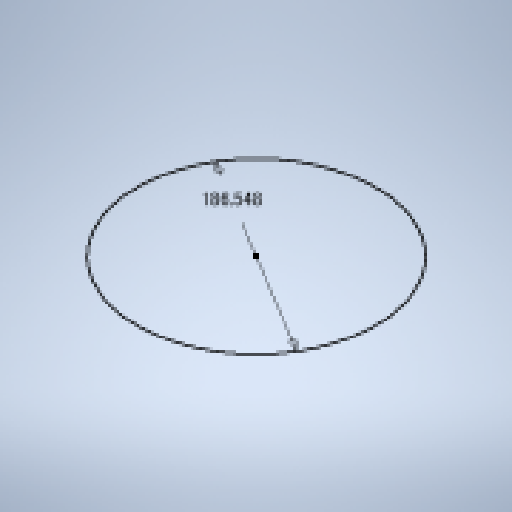
# Autodesk Inventor part: baseplate_R2toR3
Saved by Autodesk Inventor 2024.3 (Build 283343010, 343A)
## iProperties
Created: 2025-05-25
Part Number: baseplate_R2toR3
Material: アルミニウム 6061
Document SubType Name: Modeling
Designer: kshau
Density: 2.7 g/cm^3
Appearance: アルミニウム - フラット
Mass: 150.999 g
Surface Area: 394.685 cm^2
Volume: 55.9256 cm^3
Author: kshau
Autodesk Inventor part; units mm, degrees
ref_plane "YZ Plane" through (0, 0, 0) normal (1, 0, 0) x (0, 1, 0)
ref_plane "XZ Plane" through (0, 0, 0) normal (0, 1, 0) x (-1, 0, 0)
ref_plane "XY Plane" through (0, 0, 0) normal (0, 0, 1) x (1, 0, 0)
sketch "スケッチ1" plane through (0, 0, 0) normal (0, 1, 0) x (-1, 0, 0)
  circle A0 centre (0, 0) radius 86.2565
  circle A1 centre (0, 0) radius 6.25
  dimension "d0" = 172.513
  dimension "d1" = 12.5
  constraints: 2 centre point, 2 coincident
  measures "d0" diameter of A0
  measures "d1" diameter of A1
extrude "押し出し1" add sketch "スケッチ1" along normal blind 3
sketch "スケッチ2" plane through (0, 3, 0) normal (0, 1, 0) x (1, 0, 0)
  circle A0 centre (0, 0) radius 50.75
  point P0 (0, 50.75)
  point P1 (-50.75, 0)
  point P2 (0, -50.75)
  point P3 (50.75, 0)
  dimension "d4" = 101.5
  dimension "d7" = 360
  constraints: 1 coincident, 1 vertical alignment, 7 other
hole "穴1" at (0, 3, -50.75) at (-50.75, 3, 0) at (0, 3, 50.75) at (50.75, 3, 0) direction (0, -1, 0) diameter 4.3 end through all
sketch "スケッチ3" plane through (0, 3, 0) normal (0, 1, 0) x (1, 0, 0)
  line L0 (0, 0) -> (86.2565, 0)
  circle A0 centre (0, 0) radius 86.2565 projected
  circle A1 centre (0, 0) radius 6.25 projected
  line L1 (0, 0) -> (60.9926, -60.9926)
  line L2 (1.0606, -86.25) -> (-86.25, 1.0606)
  line L3 (86.25, -1.0606) -> (-1.0606, 86.25)
  point P0 (-1.0606, 86.25)
  point P1 (85.1894, 0)
  point P2 (86.25, -1.0606)
  dimension "d16" = 45
  dimension "d17" = 60.238
  constraints: 8 end point, 4 point on circle, 2 symmetric about line, 1 horizontal, 1 parallel
  measures "d16" angle of L0 L1
  measures "d17" distance between parallel lines of L1 L2
extrude "押し出し2" cut sketch "スケッチ3" against normal blind 3 contours L3 A0 L0 | L0 A0 L3 | A0 L2
sketch "スケッチ4" plane through (0, 3, 0) normal (0, 1, 0) x (1, 0, 0)
  circle A0 centre (0, 0) radius 6.25 projected
  circle A1 centre (0, 0) radius 12
  line L0 (0, 0) -> (-8.4853, -8.4853)
  line L1 (0, 0) -> (-12, 0)
  point P0 (3.1058, -11.5911)
  point P1 (11.5911, -3.1058)
  point P2 (8.4853, 8.4853)
  point P3 (-3.1058, 11.5911)
  point P4 (-11.5911, 3.1058)
  dimension "d20" = 24
  dimension "d21" = 45
  dimension "d24" = 360
  constraints: 4 end point, 2 coincident, 2 point on circle, 1 centre point, 1 horizontal, 7 other
  measures "d20" diameter of A1
  measures "d21" angle of L1 L0
hole "穴2" at (-8.4853, 3, 8.4853) at (3.1058, 3, 11.5911) at (11.5911, 3, 3.1058) at (8.4853, 3, -8.4853) at (-3.1058, 3, -11.5911) at (-11.5911, 3, -3.1058) direction (0, -1, 0) diameter 4.3 end through all
sketch "スケッチ5" plane through (0, 3, 0) normal (0, 1, 0) x (1, 0, 0)
  arc A0 (1.0606, -86.25) -> (86.25, -1.0606) centre (0, 0) ccw projected
  line L0 (14.0562, -85.1035) -> (-85.1035, 14.0562)
  arc A1 (-1.0606, 86.25) -> (-86.25, 1.0606) centre (0, 0) ccw projected
  line L1 (-86.25, 1.0606) -> (1.0606, -86.25) projected
  line L2 (-14.0562, 85.1035) -> (85.1035, -14.0562)
  line L3 (86.25, -1.0606) -> (-1.0606, 86.25) projected
  line L4 (-86.25, 1.0606) -> (-1.0606, 86.25)
  line L5 (1.0606, -86.25) -> (86.25, -1.0606)
  line L6 (-73.8926, 2.8453) -> (-2.8453, 73.8926)
  line L7 (80.9636, 4.2257) -> (2.8453, -73.8926)
  point P0 (73.8926, -2.8453)
  dimension "d33" = 10
  dimension "d34" = 10
  dimension "d35" = 7.476
  dimension "d36" = 7.476
  constraints: 12 end point, 6 point on line, 4 perpendicular, 4 point on circle, 3 coincident, 2 parallel
  measures "d33" distance between parallel lines of L1 L0
  measures "d34" distance between parallel lines of L3 L2
  measures "d35" distance between parallel lines of L4 L6
  measures "d36" distance between parallel lines of L5 L7
hole "穴3" at (-73.8926, 3, -2.8453) at (-2.8453, 3, -73.8926) at (73.8926, 3, 2.8453) at (2.8453, 3, 73.8926) direction (0, -1, 0) diameter 3.2 end through all
